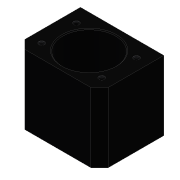
# Autodesk Inventor part: Ballnut_Support
Saved by Autodesk Inventor 2016 (Build 200138000, 138)
## iProperties
Created: 2015-07-24
Part Number: Ballnut_Support
Material: Generic
Document SubType Name: Modeling
Density: 1 g/cm^3
Appearance: Smooth - Black
Autodesk Inventor part; units mm, degrees
ref_plane "YZ Plane" through (0, 0, 0) normal (1, 0, 0) x (0, 1, 0)
ref_plane "XZ Plane" through (0, 0, 0) normal (0, 1, 0) x (-1, 0, 0)
ref_plane "XY Plane" through (0, 0, 0) normal (0, 0, 1) x (1, 0, 0)
sketch "Sketch1" plane through (0, 0, 0) normal (0, 0, 1) x (1, 0, 0)
  line L0 (-24, -18.5) -> (24, -18.5)
  line L1 (24, -18.5) -> (24, 18.5)
  line L2 (24, 18.5) -> (-24, 18.5)
  line L3 (-24, 18.5) -> (-24, -18.5)
  line L4 (-24, -18.5) -> (24, 18.5) construction
  line L5 (24, -18.5) -> (-24, 18.5) construction
  point P0 (0, 0)
  dimension "d0" = 48
  dimension "d1" = 37
  constraints: 12 end point, 2 midpoint, 2 parallel, 1 horizontal, 1 perpendicular
  measures "d0" distance of L2.end L1.end
  measures "d1" distance of L1.end L0.end
extrude "Extrusion1" add sketch "Sketch1" along normal mid plane 40
chamfer "Chamfer1" distance 5 angle 45 2 edges at (24, -18.5, 0) (-24, -18.5, 0)
sketch "Sketch2" plane through (0, 0, 20) normal (0, 0, 1) x (1, 0, 0)
  line L0 (24, 18.5) -> (-24, 18.5) projected
  point P0 (0, 0)
  point P1 (0, -0.5)
  point P2 (0, 18.5)
  dimension "d7" = 19
  constraints: 1 midpoint, 1 vertical alignment
  measures "d7" distance from line of L0 point (0, -0.5)
hole "Hole1" at (0, -0.5, 20) direction (0, 0, -1) diameter 30.5 end through all
chamfer "Chamfer2" distance 0.5 angle 45 2 edges at (0, 14.75, 20) (0, 14.75, -20)
sketch "Sketch3" plane through (-24, 18.5, 20) normal (0, 1, 0) x (1, 0, 0)
  line L0 (44, 7.5) -> (4, 7.5)
  line L1 (4, 7.5) -> (4, 32.5)
  line L2 (4, 32.5) -> (44, 32.5)
  line L3 (44, 32.5) -> (44, 7.5)
  line L4 (44, 7.5) -> (4, 32.5) construction
  line L5 (4, 7.5) -> (44, 32.5) construction
  point P0 (24, 20)
  dimension "d18" = 25
  dimension "d19" = 40
  constraints: 12 end point, 2 midpoint, 2 parallel, 1 horizontal, 1 perpendicular
  measures "d18" distance of L0.end L1.end
  measures "d19" distance of L1.end L2.end
hole "Hole2" at (-20, 18.5, -12.5) at (-20, 18.5, 12.5) at (20, 18.5, -12.5) at (20, 18.5, 12.5) direction (0, -1, 0) diameter 3.242 depth 12 tip angle 118 thread size "M4x0.7" designation "M4" class "6H" standard "ISO Metric profile"
sketch "Sketch4" plane through (0, 0, 20) normal (0, 0, 1) x (1, 0, 0)
  circle A0 centre (0, -0.5) radius 20 construction
  circle A1 centre (0, -0.5) radius 15.25 projected
  point P0 (0, 0)
  point P1 (-17.3205, 9.5)
  point P2 (-17.3205, -10.5)
  point P3 (17.3205, -10.5)
  point P4 (17.3205, 9.5)
  dimension "d27" = 20
  dimension "d28" = 40
  constraints: 4 point on circle, 2 vertical alignment, 1 centre point, 1 concentric, 1 horizontal alignment
  measures "d27" distance of A0.end A0.start
  measures "d28" diameter of A0
hole "Hole4" at (-17.3205, 9.5, 20) at (-17.3205, -10.5, 20) at (17.3205, -10.5, 20) at (17.3205, 9.5, 20) direction (0, 0, -1) diameter 3.242 depth 10 tip angle 118 thread size "M4x0.7" class "6H" standard "ISO Metric profile"
body "Solid1"
